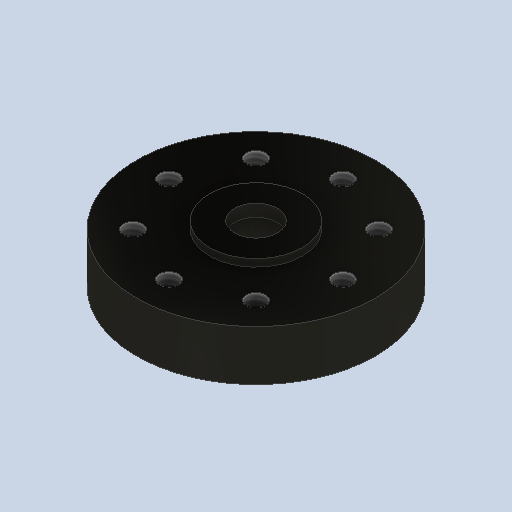
# Autodesk Inventor part: Servo_horn_Top
Saved by Autodesk Inventor 2023 (Build 270158000, 158)
## iProperties
Created: 2022-09-18
Part Number: Servo_horn_Top
Material: 일반
Document SubType Name: Modeling
Designer: 박동준
Density: 1 g/cm^3
Appearance: 기본값
품번: 8
Author: 박동준
Autodesk Inventor part; units mm, degrees
ref_plane "YZ Plane" through (0, 0, 0) normal (1, 0, 0) x (0, 1, 0)
ref_plane "XZ Plane" through (0, 0, 0) normal (0, 1, 0) x (-1, 0, 0)
ref_plane "XY Plane" through (0, 0, 0) normal (0, 0, 1) x (1, 0, 0)
sketch "스케치1" plane through (0, 0, 0) normal (0, 0, 1) x (1, 0, 0)
  line L0 (0, 2.8205) -> (0, -2.8205)
  line L1 (1.75, 3) -> (1.75, 2)
  line L2 (1.75, 2) -> (2.925, 2)
  line L3 (2.925, 2) -> (2.925, -2)
  line L4 (2.925, -2) -> (4.45, -2)
  line L5 (4.45, -2) -> (4.45, -1.7)
  line L6 (4.45, -1.7) -> (9.75, -1.7)
  line L7 (9.75, -1.7) -> (9.75, 2.4)
  line L8 (9.75, 2.4) -> (3.8, 2.4)
  line L9 (3.8, 2.4) -> (3.8, 3)
  line L10 (3.8, 3) -> (1.75, 3)
  point P0 (0, 0)
  point P1 (0, 0)
  point P2 (2.925, 0)
  dimension "d0" = 0.3
  dimension "d1" = 1.75
  dimension "d2" = 2.925
  dimension "d3" = 3.8
  dimension "d4" = 4.1
  dimension "d5" = 0.6
  dimension "d6" = 4.45
  dimension "d7" = 9.75
  dimension "d8" = 1
  constraints: 22 end point, 7 perpendicular, 3 midpoint, 2 vertical, 1 coincident, 1 horizontal alignment, 1 parallel
  measures "d0" distance of L4.end L5.end
  measures "d1" distance between parallel lines of L1 L0
  measures "d2" distance between parallel lines of L3 L0
  measures "d3" distance between parallel lines of L0 L9
  measures "d4" distance of L6.end L7.end
  measures "d5" distance between parallel lines of L10 L8
  measures "d6" distance between parallel lines of L0 L5
  measures "d7" distance between parallel lines of L7 L0
  measures "d8" distance of L1.start L1.end
revolve "회전1" add sketch "스케치1" angle 360 about axis through (0, 2.8205, 0) along (0, -1, 0)
sketch "스케치2" plane through (0, 2.4, 0) normal (0, 1, 0) x (1, 0, 0)
  circle A0 centre (0, 0) radius 3.8 projected
  circle A1 centre (0, 0) radius 9.75 projected
  circle A2 centre (0, 0) radius 1.75 projected
  circle A3 centre (0, 0) radius 3.8 projected
  circle A4 centre (0, 0) radius 1.75 projected
  circle A5 centre (0, 0) radius 3.8 projected
  point P0 (0, 0)
  point P1 (7.1, 0)
  point P2 (5.0205, 5.0205)
  point P3 (0, 7.1)
  point P4 (-5.0205, 5.0205)
  point P5 (-7.1, 0)
  point P6 (-5.0205, -5.0205)
  point P7 (0, -7.1)
  point P8 (5.0205, -5.0205)
  dimension "d10" = 7.1
  dimension "d13" = 360
  constraints: 9 other
  measures "d10" distance of point (7.1, 0) point (0, 0)
hole "구멍1" at (7.1, 2.4, 0) at (5.0205, 2.4, -5.0205) at (0, 2.4, -7.1) at (-5.0205, 2.4, -5.0205) at (-7.1, 2.4, 0) at (-5.0205, 2.4, 5.0205) at (0, 2.4, 7.1) at (5.0205, 2.4, 5.0205) direction (0, -1, 0) diameter 1.567 end through all thread size "M2x0.4" class "6H" standard "ISO Metric profile"
